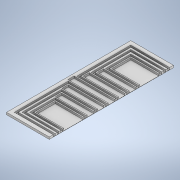
# Autodesk Inventor part: wire_holder_half1
Saved by Autodesk Inventor 2021 (Build 250183000, 183)
## iProperties
Created: 2021-02-03
Part Number: wire_holder_half1
Material: Generic
Document SubType Name: Modeling
Designer: User
Density: 1 g/cm^3
Appearance: Default
Author: User
Autodesk Inventor part; units mm, degrees
ref_plane "YZ Plane" through (0, 0, 0) normal (1, 0, 0) x (0, 1, 0)
ref_plane "XZ Plane" through (0, 0, 0) normal (0, 1, 0) x (-1, 0, 0)
ref_plane "XY Plane" through (0, 0, 0) normal (0, 0, 1) x (1, 0, 0)
sketch "Sketch1" plane through (0, 0, 0) normal (0, 1, 0) x (-1, 0, 0)
  line L0 (381.5779, 150) -> (481.5779, 150)
  line L1 (481.5779, 150) -> (481.5779, 11)
  line L2 (381.5779, 145) -> (476.5779, 145)
  line L3 (476.5779, 145) -> (476.5779, 16)
  line L4 (476.5779, 16) -> (381.5779, 16)
  line L5 (481.5779, 11) -> (381.5779, 11)
  line L6 (381.5779, 135) -> (466.5779, 135)
  line L7 (381.5779, 140) -> (471.5779, 140)
  line L8 (466.5779, 135) -> (466.5779, 43)
  line L9 (466.5779, 43) -> (381.5779, 43)
  line L10 (471.5779, 140) -> (471.5779, 38)
  line L11 (471.5779, 38) -> (381.5779, 38)
  line L12 (381.5779, 125) -> (456.5779, 125)
  line L13 (456.5779, 125) -> (456.5779, 70)
  line L14 (456.5779, 70) -> (381.5779, 70)
  line L15 (381.5779, 130) -> (461.5779, 130)
  line L16 (461.5779, 130) -> (461.5779, 65)
  line L17 (461.5779, 65) -> (381.5779, 65)
  line L18 (381.5779, -11) -> (481.5779, -11)
  line L19 (481.5779, -11) -> (481.5779, -150)
  line L20 (481.5779, -150) -> (381.5779, -150)
  line L21 (381.5779, -16) -> (476.5779, -16)
  line L22 (476.5779, -16) -> (476.5779, -145)
  line L23 (476.5779, -145) -> (381.5779, -145)
  line L24 (381.5779, -38) -> (471.5779, -38)
  line L25 (471.5779, -38) -> (471.5779, -140)
  line L26 (471.5779, -140) -> (381.5779, -140)
  line L27 (381.5779, -43) -> (466.5779, -43)
  line L28 (466.5779, -43) -> (466.5779, -135)
  line L29 (466.5779, -135) -> (381.5779, -135)
  line L30 (381.5779, -65) -> (461.5779, -65)
  line L31 (461.5779, -65) -> (461.5779, -130)
  line L32 (381.5779, -70) -> (456.5779, -70)
  line L33 (456.5779, -70) -> (456.5779, -125)
  line L34 (456.5779, -125) -> (381.5779, -125)
  line L35 (461.5779, -130) -> (381.5779, -130)
  line L36 (491.5779, 160) -> (491.5779, -160)
  line L37 (491.5779, -160) -> (381.5779, -160)
  line L38 (381.5779, 160) -> (491.5779, 160)
  line L39 (381.5779, -212.9987) -> (381.5779, 354.6855) construction
  line L40 (381.5779, -160) -> (381.5779, 160)
  line L41 (381.5779, 122) -> (453.5779, 122)
  line L42 (453.5779, 122) -> (453.5779, 73)
  line L43 (453.5779, 73) -> (381.5779, 73)
  line L44 (381.5779, 73) -> (381.5779, 122)
  line L45 (463.5779, 62) -> (381.5779, 62)
  line L46 (381.5779, 62) -> (381.5779, 46)
  line L47 (381.5779, 46) -> (463.5779, 46)
  line L48 (463.5779, 46) -> (463.5779, 62)
  line L49 (381.5779, 8) -> (485.5779, 8)
  line L50 (485.5779, 8) -> (485.5779, -8)
  line L51 (485.5779, -8) -> (381.5779, -8)
  line L52 (381.5779, -8) -> (381.5779, 8)
  line L53 (473.5779, 35) -> (381.5779, 35)
  line L54 (381.5779, 35) -> (381.5779, 19)
  line L55 (381.5779, 19) -> (473.5779, 19)
  line L56 (473.5779, 19) -> (473.5779, 35)
  line L57 (473.5779, -19) -> (381.5779, -19)
  line L58 (381.5779, -19) -> (381.5779, -35)
  line L59 (381.5779, -35) -> (473.5779, -35)
  line L60 (473.5779, -35) -> (473.5779, -19)
  line L61 (463.5779, -46) -> (381.5779, -46)
  line L62 (381.5779, -46) -> (381.5779, -62)
  line L63 (381.5779, -62) -> (463.5779, -62)
  line L64 (463.5779, -62) -> (463.5779, -46)
  line L65 (453.5779, -73) -> (381.5779, -73)
  line L66 (381.5779, -73) -> (381.5779, -122)
  line L67 (381.5779, -122) -> (453.5779, -122)
  line L68 (453.5779, -122) -> (453.5779, -73)
  dimension "d3" = 5
  dimension "d4" = 5
  dimension "d7" = 5
  dimension "d8" = 5
  dimension "d9" = 5
  dimension "d10" = 5
  dimension "d14" = 5
  dimension "d16" = 5
  dimension "d18" = 5
  dimension "d19" = 5
  dimension "d20" = 22
  dimension "d21" = 5
  dimension "d22" = 5
  dimension "d30" = 5
  dimension "d31" = 5
  dimension "d32" = 5
  dimension "d36" = 5
  dimension "d37" = 5
  dimension "d38" = 5
  dimension "d40" = 5
  dimension "d43" = 5
  dimension "d44" = 5
  dimension "d45" = 5
  dimension "d48" = 5
  dimension "d49" = 5
  dimension "d57" = 10
  dimension "d63" = 110
  dimension "d64" = 3
  dimension "d65" = 3
  dimension "d66" = 3
  dimension "d67" = 3
  dimension "d68" = 3
  dimension "d69" = 3
  dimension "d70" = 6
  dimension "d71" = 3
  dimension "d72" = 3
  dimension "d73" = 3
  dimension "d74" = 3
  dimension "d75" = 3
  dimension "d76" = 3
  dimension "d77" = 3
  dimension "d78" = 3
  dimension "d79" = 3
  dimension "d80" = 3
  dimension "d81" = 3
  dimension "d82" = 3
  dimension "d83" = 3
  dimension "d84" = 3
  constraints: 134 end point, 26 perpendicular, 25 horizontal, 19 parallel, 4 vertical, 39 other
  measures "d3" distance between parallel lines of L0 L2
  measures "d4" distance between parallel lines of L3 L1
  measures "d7" distance between parallel lines of L5 L4
  measures "d8" distance between parallel lines of L8 L10
  measures "d9" distance between parallel lines of L7 L6
  measures "d10" distance between parallel lines of L10 L3
  measures "d14" distance between parallel lines of L11 L9
  measures "d16" distance between parallel lines of L6 L15
  measures "d18" distance between parallel lines of L15 L12
  measures "d19" distance between parallel lines of L16 L8
  measures "d20" distance between parallel lines of L9 L17
  measures "d21" distance between parallel lines of L16 L13
  measures "d22" distance between parallel lines of L17 L14
  measures "d30" distance between parallel lines of L21 L18
  measures "d31" distance between parallel lines of L22 L19
  measures "d32" distance between parallel lines of L20 L23
  measures "d36" distance between parallel lines of L28 L25
  measures "d37" distance between parallel lines of L25 L22
  measures "d38" distance between parallel lines of L24 L27
  measures "d40" distance between parallel lines of L26 L29
  measures "d43" distance between parallel lines of L30 L32
  measures "d44" distance between parallel lines of L33 L31
  measures "d45" distance between parallel lines of L31 L28
  measures "d48" distance between parallel lines of L35 L34
  measures "d49" distance between parallel lines of L29 L35
  measures "d57" distance between parallel lines of L36 L19
  measures "d64" distance between parallel lines of L12 L41
  measures "d65" distance between parallel lines of L13 L42
  measures "d66" distance between parallel lines of L43 L14
  measures "d67" distance between parallel lines of L17 L45
  measures "d68" distance between parallel lines of L48 L8
  measures "d69" distance between parallel lines of L47 L9
  measures "d70" distance between parallel lines of L36 L50
  measures "d71" distance between parallel lines of L18 L51
  measures "d72" distance between parallel lines of L5 L49
  measures "d73" distance between parallel lines of L11 L53
  measures "d74" distance between parallel lines of L55 L4
  measures "d75" distance between parallel lines of L56 L3
  measures "d76" distance between parallel lines of L60 L22
  measures "d77" distance between parallel lines of L21 L57
  measures "d78" distance between parallel lines of L59 L24
  measures "d79" distance between parallel lines of L27 L61
  measures "d80" distance between parallel lines of L63 L30
  measures "d81" distance between parallel lines of L28 L64
  measures "d82" distance between parallel lines of L32 L65
  measures "d83" distance between parallel lines of L33 L68
  measures "d84" distance between parallel lines of L67 L34
extrude "Extrusion1" add sketch "Sketch1" along normal blind 5 contours L40 L38 L36 L37 L20 L19 L18 L51 L50 L49 L5 L1 L0 | L2 L3 L4 L40 L55 L56 L53 L11 L10 L7 | L6 L8 L9 L40 L47 L48 L45 L17 L16 L15 | L12 L13 L14 L40 L43 L42 L41 | L40 L26 L25 L24 L59 L60 L57 L21 L22 L23 | L40 L35 L31 L30 L63 L64 L61 L27 L28 L29 | L40 L67 L68 L65 L32 L33 L34
sketch "Sketch2" plane through (-491.5779, 0, 160) normal (0, 0, 1) x (1, 0, 0)
  line L0 (0, 0) -> (0, 5) projected
  line L1 (0, 0) -> (110, 0)
  line L2 (110, 0) -> (110, -0.5)
  line L3 (110, -0.5) -> (0, -0.5)
  line L4 (0, -0.5) -> (0, 0)
  point P0 (491.5779, 0)
  dimension "d87" = 0.5
  constraints: 8 end point, 2 parallel, 1 horizontal, 1 perpendicular
  measures "d87" distance of L1.end L2.end
extrude "Extrusion2" add sketch "Sketch2" against normal blind 320
equation "\"d3\" = d25"
equation "\"d4\" = d25"
equation "\"d7\" = d25"
equation "\"d8\" = d25"
equation "\"d9\" = d25"
equation "\"d10\" = d26"
equation "\"d14\" = d25"
equation "\"d16\" = d26"
equation "\"d18\" = d25"
equation "\"d19\" = d25"
equation "\"d20\" = d28"
equation "\"d21\" = d25"
equation "\"d22\" = d25"
equation "\"d30\" = d51"
equation "\"d31\" = d51"
equation "\"d32\" = d51"
equation "\"d36\" = d51"
equation "\"d37\" = d53"
equation "\"d38\" = d51"
equation "\"d40\" = d51"
equation "\"d43\" = d51"
equation "\"d44\" = d51"
equation "\"d45\" = d53"
equation "\"d48\" = d51"
equation "\"d49\" = d53"
equation "\"d25\" = 5"
equation "\"d26\" = 5"
equation "\"d28\" = -1.2 * d25 + 0.2 * d29"
equation "\"d51\" = 5"
equation "\"d53\" = 5"
equation "\"d54\" = -1.2 * d51 + 0.2 * d55"
equation "\"d29\" = 140"
equation "\"d55\" = 140"
body "Solid1"
